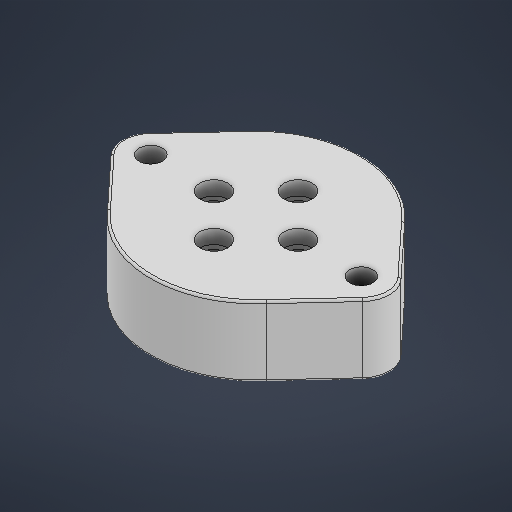
# Autodesk Inventor part: neck
Saved by Autodesk Inventor 2026 (Build 300175000, 175)
## iProperties
Created: 2025-04-16
Part Number: neck
Material: Generic
Document SubType Name: Modeling
Designer: Elizabeth
Density: 1 g/cm^3
Appearance: Default
Author: Elizabeth
Autodesk Inventor part; units mm, degrees
ref_plane "YZ Plane" through (0, 0, 0) normal (1, 0, 0) x (0, 1, 0)
ref_plane "XZ Plane" through (0, 0, 0) normal (0, 1, 0) x (-1, 0, 0)
ref_plane "XY Plane" through (0, 0, 0) normal (0, 0, 1) x (1, 0, 0)
sketch "Sketch1" plane through (0, 0, 0) normal (0, 1, 0) x (-1, 0, 0)
  circle A0 centre (0, 0) radius 15
  circle A1 centre (0, 0) radius 8.5
  circle A2 centre (15, 0) radius 4
  circle A3 centre (-15, 0) radius 4
  line L0 (10.6066, -10.6066) -> (17.9306, -2.7224)
  line L1 (-10.6066, -10.6066) -> (-17.9306, -2.7224)
  line L2 (10.6066, 10.6066) -> (17.9306, 2.7224)
  line L3 (-10.6066, 10.6066) -> (-17.9306, 2.7224)
  line L4 (16.6, -2.7713) -> (13.4, -2.7713)
  line L5 (13.4, -2.7713) -> (11.8, 0)
  line L6 (11.8, 0) -> (13.4, 2.7713)
  line L7 (13.4, 2.7713) -> (16.6, 2.7713)
  line L8 (16.6, 2.7713) -> (18.2, 0)
  line L9 (18.2, 0) -> (16.6, -2.7713)
  line L10 (15, -2.7713) -> (15, 2.7713)
  line L11 (11.8, 0) -> (15, 0)
  line L12 (-13.4, -2.7713) -> (-16.6, -2.7713)
  line L13 (-16.6, -2.7713) -> (-18.2, 0)
  line L14 (-18.2, 0) -> (-16.6, 2.7713)
  line L15 (-16.6, 2.7713) -> (-13.4, 2.7713)
  line L16 (-13.4, 2.7713) -> (-11.8, 0)
  line L17 (-11.8, 0) -> (-13.4, -2.7713)
  line L18 (-15, -2.7713) -> (-15, 2.7713)
  line L19 (-18.2, 0) -> (-15, 0)
  circle A4 centre (0, 0) radius 6
  circle A5 centre (0, -6) radius 1.2
  circle A6 centre (-6, 0) radius 1.2
  circle A7 centre (0, 6) radius 1.2
  circle A8 centre (6, 0) radius 1.2
  circle A9 centre (15, 0) radius 1.65
  circle A10 centre (-15, 0) radius 1.65
  point P0 (-11.3582, -9.7975)
  point P1 (11.3582, -9.7975)
  point P2 (11.3582, 9.7976)
  point P3 (-11.3582, 9.7976)
  dimension "d20" = 8
  dimension "d22" = 3.2
  dimension "d27" = 3.2
  dimension "d28" = 3.2
  dimension "d29" = 120
  dimension "d30" = 3.2
  dimension "d31" = 120
  dimension "d34" = 12
  dimension "d35" = 2.4
  dimension "d36" = 2.4
  dimension "d37" = 2.4
  dimension "d38" = 2.4
  dimension "d43" = 3.3
  dimension "d44" = 3.3
  constraints: 40 end point, 10 centre point, 7 point on circle, 6 midpoint, 4 coincident, 4 horizontal, 4 other
  measures "d20" diameter of A3
  measures "d22" distance of L4.start L4.end
  measures "d27" distance of L12.start L12.end
  measures "d28" distance of L12.end L13.end
  measures "d29" angle of L12 L13
  measures "d30" distance of L13.end L14.end
  measures "d31" angle of L13 L14
  measures "d34" diameter of A4
  measures "d35" diameter of A5
  measures "d36" diameter of A6
  measures "d37" diameter of A7
  measures "d38" diameter of A8
  measures "d43" diameter of A9
  measures "d44" diameter of A10
extrude "Extrusion1" add sketch "Sketch1" along normal blind 10 contours L2 A0 A2 L0 L1 A3 L3 | A0 L2 | L3 A0 | L2 A2 A0 | A0 A3 L3 | A2 A0 L4 L9 L8 L7 | A0 L7 L6 L5 L4 A2 | A3 A0 L12 L17 L16 L15 | A0 L15 L14 L13 L12 A3 | L7 L10 A9 A0 | A0 A9 L11 L6 L7 | A2 L0 A0 | L15 L16 L17 L12 A0 A10 | A0 A10 L18 L15 | A3 A0 L1 | A9 L10 A0 | A0 L11 A9 | L7 L8 L9 L4 L10 A9 | A0 L0 | L4 L5 L11 A9 A0 | A0 A9 L10 L4 | A10 A0 | A0 L18 A10 | L18 A10 L19 L14 L15 | L1 A0 | L10 A9 A0 | L10 A9 | A0 A9 L11 | A0 A10 L18 | L19 A10 L18 | L18 A10 L19 | L12 L18 A10 A0 | L18 L12 L13 L19 A10 | A1 | A4 A8 | A4 A8 | A8 A4 A5 A6 A7 | A7 A4 | A4 A7 | A5 A4 | A4 A5 | A6 A4 | A4 A6
extrude "Extrusion2" cut sketch "Sketch1" along normal blind 2.5 contours L7 L10 A9 A0 | A0 A9 L11 L6 L7 | L15 L16 L17 L12 A0 A10 | A0 A10 L18 L15 | A9 L10 A0 | A0 L11 A9 | L7 L8 L9 L4 L10 A9 | L4 L5 L11 A9 A0 | A0 A9 L10 L4 | A10 A0 | A0 L18 A10 | L18 A10 L19 L14 L15 | L10 A9 A0 | L10 A9 | A0 A9 L11 | A0 A10 L18 | L19 A10 L18 | L18 A10 L19 | L12 L18 A10 A0 | L18 L12 L13 L19 A10 | A1 | A4 A8 | A4 A8 | A8 A4 A5 A6 A7 | A7 A4 | A4 A7 | A5 A4 | A4 A5 | A6 A4 | A4 A6
extrude "Extrusion3" cut sketch "Sketch1" along normal blind 10 contours A9 L10 A0 | A0 L11 A9 | A10 A0 | A0 L18 A10 | L10 A9 A0 | L10 A9 | A0 A9 L11 | A0 A10 L18 | L19 A10 L18 | L18 A10 L19 | A4 A8 | A4 A8 | A7 A4 | A4 A7 | A5 A4 | A4 A5 | A6 A4 | A4 A6
fillet "Fillet1" radius 0.3 16 edges at (0, 0, -15) (-19, 0, 0) (-14.6444, 0, 6.26) (-14.6444, 0, -6.26) (0, 0, 15) (19, 0, 0) (14.6444, 0, -6.26) (14.6444, 0, 6.26) (-19, 10, 0) (-14.6444, 10, 6.26) (-14.6444, 10, -6.26) (0, 10, -15) (0, 10, 15) (19, 10, 0) (14.6444, 10, 6.26) (14.6444, 10, -6.26)
sketch "Sketch2" plane through (0, 10, 0) normal (0, 1, 0) x (1, 0, 0)
  circle A0 centre (-6, 0) radius 1.2 projected
  circle A1 centre (-6, 0) radius 2
  circle A2 centre (0, 6) radius 1.2 projected
  circle A3 centre (0, 6) radius 2
  circle A4 centre (6, 0) radius 1.2 projected
  circle A5 centre (6, 0) radius 2
  circle A6 centre (0, -6) radius 1.2 projected
  circle A7 centre (0, -6) radius 2
  point P0 (0, 0)
  dimension "d48" = 4
  dimension "d49" = 4
  dimension "d50" = 4
  dimension "d51" = 4
  constraints: 4 centre point, 4 coincident
  measures "d48" diameter of A1
  measures "d49" diameter of A3
  measures "d50" diameter of A5
  measures "d51" diameter of A7
extrude "Extrusion5" cut sketch "Sketch2" against normal blind 2 contours A0 | A1 | A2 | A3 | A4 | A5 | A6 | A7
body "Solid1"
